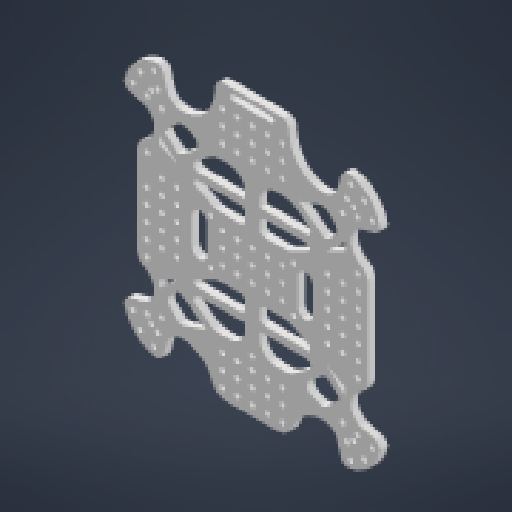
# Autodesk Inventor part: bottom
Saved by Autodesk Inventor 2023 (Build 270158000, 158)
## iProperties
Created: 2022-05-28
Part Number: bottom
Material: Generic
Document SubType Name: Modeling
Designer: vibhu
Density: 1 g/cm^3
Appearance: Default
Author: vibhu
Autodesk Inventor part; units mm, degrees
ref_plane "YZ Plane" through (0, 0, 0) normal (1, 0, 0) x (0, 1, 0)
ref_plane "XZ Plane" through (0, 0, 0) normal (0, 1, 0) x (-1, 0, 0)
ref_plane "XY Plane" through (0, 0, 0) normal (0, 0, 1) x (1, 0, 0)
sketch "Base Sketch With Dimensions" plane through (0, 0, 0) normal (0, 0, 1) x (1, 0, 0)
  circle A0 centre (74.1421, 4.1421) radius 1.75
  circle A1 centre (60, -10) radius 1.75
  circle A2 centre (69.6593, -7.4118) radius 1.75
  circle A3 centre (79.3185, -4.8236) radius 1.75
  circle A4 centre (65.1764, 9.3185) radius 1.75
  circle A5 centre (62.5882, -0.3407) radius 1.75
  line L0 (65.1764, 9.3185) -> (60, -10) construction
  line L1 (60, -10) -> (74.1421, 4.1421) construction
  line L2 (60, -10) -> (79.3185, -4.8236) construction
  circle A6 centre (67.0711, -2.9289) radius 1.75
  circle A7 centre (-74.1421, -144.1421) radius 1.75
  circle A8 centre (-60, -130) radius 1.75
  circle A9 centre (-69.6593, -132.5882) radius 1.75
  circle A10 centre (-79.3185, -135.1764) radius 1.75
  circle A11 centre (-65.1764, -149.3185) radius 1.75
  circle A12 centre (-62.5882, -139.6593) radius 1.75
  line L3 (-65.1764, -149.3185) -> (-60, -130) construction
  line L4 (-60, -130) -> (-74.1421, -144.1421) construction
  line L5 (-60, -130) -> (-79.3185, -135.1764) construction
  circle A13 centre (-67.0711, -137.0711) radius 1.75
  circle A14 centre (-74.1421, 4.1421) radius 1.75
  circle A15 centre (-60, -10) radius 1.75
  circle A16 centre (-62.5882, -0.3407) radius 1.75
  circle A17 centre (-65.1764, 9.3185) radius 1.75
  circle A18 centre (-79.3185, -4.8236) radius 1.75
  circle A19 centre (-69.6593, -7.4118) radius 1.75
  line L6 (-79.3185, -4.8236) -> (-60, -10) construction
  line L7 (-60, -10) -> (-74.1421, 4.1421) construction
  line L8 (-60, -10) -> (-65.1764, 9.3185) construction
  circle A20 centre (-67.0711, -2.9289) radius 1.75
  circle A21 centre (74.1421, -144.1421) radius 1.75
  circle A22 centre (60, -130) radius 1.75
  circle A23 centre (62.5882, -139.6593) radius 1.75
  circle A24 centre (65.1764, -149.3185) radius 1.75
  circle A25 centre (79.3185, -135.1764) radius 1.75
  circle A26 centre (69.6593, -132.5882) radius 1.75
  line L9 (79.3185, -135.1764) -> (60, -130) construction
  line L10 (60, -130) -> (74.1421, -144.1421) construction
  line L11 (60, -130) -> (65.1764, -149.3185) construction
  circle A27 centre (67.0711, -137.0711) radius 1.75
  line L12 (-22.5, 0) -> (22.5, 0) construction
  line L13 (22.5, 0) -> (22.5, -140) construction
  line L14 (22.5, -140) -> (-22.5, -140) construction
  line L15 (-22.5, -140) -> (-22.5, 0) construction
  line L16 (-67.5, -35) -> (-42.5, -35) construction
  line L17 (-42.5, -35) -> (-42.5, -105) construction
  line L18 (-42.5, -105) -> (-67.5, -105) construction
  line L19 (-67.5, -105) -> (-67.5, -35) construction
  line L20 (42.5, -35) -> (67.5, -35) construction
  line L21 (67.5, -35) -> (67.5, -105) construction
  line L22 (67.5, -105) -> (42.5, -105) construction
  line L23 (42.5, -105) -> (42.5, -35) construction
  line L24 (-42.5, -70) -> (-22.5, -70) construction
  line L25 (22.5, -70) -> (42.5, -70) construction
  line L26 (-60, -10) -> (-60, -130) construction
  line L27 (60, -130) -> (-60, -130) construction
  arc A28 (84.5585, -5.3225) -> (64.6775, 14.5585) centre (60, -10) ccw
  line L28 (58.9124, 10.9409) -> (54.7169, -4.7169)
  line L29 (80.9409, -11.0876) -> (65.2831, -15.2831)
  arc A29 (64.6775, 14.5585) -> (58.9124, 10.9409) centre (63.742, 9.6468) ccw
  arc A30 (80.9409, -11.0876) -> (84.5585, -5.3225) centre (79.6468, -6.258) ccw
  line L30 (0, 57.9218) -> (0, -169.8921) construction
  line L31 (161.6421, -70) -> (-111.9125, -70) construction
  arc A31 (-64.6775, 14.5585) -> (-84.5585, -5.3225) centre (-60, -10) ccw
  line L32 (-58.9124, 10.9409) -> (-54.7169, -4.7169)
  line L33 (-80.9409, -11.0876) -> (-65.2831, -15.2831)
  arc A32 (-58.9124, 10.9409) -> (-64.6775, 14.5585) centre (-63.742, 9.6468) ccw
  arc A33 (-84.5585, -5.3225) -> (-80.9409, -11.0876) centre (-79.6468, -6.258) ccw
  arc A34 (64.6775, -154.5585) -> (84.5585, -134.6775) centre (60, -130) ccw
  line L34 (58.9124, -150.9409) -> (54.7169, -135.2831)
  line L35 (80.9409, -128.9124) -> (65.2831, -124.7169)
  arc A35 (58.9124, -150.9409) -> (64.6775, -154.5585) centre (63.742, -149.6468) ccw
  arc A36 (84.5585, -134.6775) -> (80.9409, -128.9124) centre (79.6468, -133.742) ccw
  arc A37 (-64.6775, -154.5585) -> (-58.9124, -150.9409) centre (-63.742, -149.6468) ccw
  line L36 (-58.9124, -150.9409) -> (-54.7169, -135.2831)
  arc A38 (-84.5585, -134.6775) -> (-64.6775, -154.5585) centre (-60, -130) ccw
  arc A39 (-80.9409, -128.9124) -> (-84.5585, -134.6775) centre (-79.6468, -133.742) ccw
  line L37 (-80.9409, -128.9124) -> (-65.2831, -124.7169)
  line L38 (54.7169, -4.7169) -> (65.2831, -15.2831) construction
  line L39 (-65.2831, -15.2831) -> (-65.2831, -124.7169)
  line L40 (65.2831, -124.7169) -> (65.2831, -15.2831)
  line L41 (-54.7169, -4.7169) -> (54.7169, -4.7169)
  line L42 (-54.7169, -135.2831) -> (54.7169, -135.2831)
  point P0 (-42.5, -70)
  point P1 (0, -130)
  point P2 (0, -140)
  point P3 (-60, -70)
  point P4 (0, 0)
  point P5 (0, 0)
  point P6 (-67.5, -70)
  point P7 (85, -10)
  point P8 (60, 15)
  point P9 (42.5, -70)
  dimension "d0" = 3.5
  dimension "d1" = 30
  dimension "d2" = 30
  dimension "d3" = 20
  dimension "d5" = 30
  dimension "d6" = 30
  dimension "d9" = 30
  dimension "d10" = 30
  dimension "d13" = 30
  dimension "d14" = 30
  dimension "d16" = 45
  dimension "d17" = 140
  dimension "d18" = 25
  dimension "d19" = 70
  dimension "d23" = 135
  dimension "d25" = 135
  dimension "d29" = 20
  dimension "d30" = 120
  dimension "d32" = 120
  dimension "d40" = 25
  dimension "d41" = 5
  constraints: 86 end point, 40 centre point, 28 equal radius, 27 symmetric about line, 26 point on circle, 25 midpoint, 18 coincident, 14 equal length, 10 horizontal alignment, 9 parallel, 7 perpendicular, 5 point on line, 4 horizontal, 4 tangent, 4 vertical alignment, 3 vertical, 10 other
  measures "d0" diameter of A4
  measures "d1" angle of L1 L0
  measures "d2" angle of L2 L1
  measures "d3" distance of L0.end L2.end
  measures "d5" angle of L4 L3
  measures "d6" angle of L5 L4
  measures "d9" angle of L7 L6
  measures "d10" angle of L8 L7
  measures "d13" angle of L10 L9
  measures "d14" angle of L11 L10
  measures "d16" distance of L13.end L14.end
  measures "d17" distance of L12.end L13.end
  measures "d18" distance of L16.start L16.end
  measures "d19" distance of L18.end L16.start
  measures "d23" angle of L26 L4
  measures "d25" angle of L26 L7
  measures "d29" distance between parallel lines of L15 L17
  measures "d30" distance of point (60, -10) point (-60, -10)
  measures "d32" distance of L6.end L3.end
  measures "d40" radius of A28
  measures "d41" radius of A29
extrude "Extrusion1" add sketch "Base Sketch With Dimensions" along normal blind 5
fillet "Fillet1" radius 10 8 edges at (54.7169, -135.2831, 2.5) (-54.7169, -135.2831, 2.5) (-65.2831, -124.7169, 2.5) (-65.2831, -15.2831, 2.5) (54.7169, -4.7169, 2.5) (-54.7169, -4.7169, 2.5) (65.2831, -15.2831, 2.5) (65.2831, -124.7169, 2.5)
sketch "Sketch3" plane through (0, 0, 0) normal (0, 0, -1) x (-1, 0, 0)
  circle A0 centre (70, -50) radius 1.75
  line L0 (0, 0) -> (-18.5117, 0) construction
  line L1 (0, 0) -> (0, -12.0208) construction
  line L2 (-65.2831, -117.0436) -> (-65.2831, -22.9564) construction
  line L3 (-47.0436, -4.7169) -> (47.0436, -4.7169) construction
  line L4 (84.7487, 0.6066) -> (70.6066, 14.7487) construction
  line L5 (-70.6066, 14.7487) -> (-84.7487, 0.6066) construction
  line L6 (-84.7487, -140.6066) -> (-70.6066, -154.7487) construction
  line L7 (70.6066, -154.7487) -> (84.7487, -140.6066) construction
  line L8 (-65.2831, -22.9564) -> (-65.2831, -117.0436) construction
  line L9 (-84.7487, 0.6066) -> (-70.6066, 14.7487) construction
  circle A1 centre (20, -150) radius 1.75
  circle A2 centre (10, -150) radius 1.75
  circle A3 centre (0, -150) radius 1.75
  circle A4 centre (-10, -150) radius 1.75
  circle A5 centre (-20, -150) radius 1.75
  circle A6 centre (20, -140) radius 1.75
  circle A7 centre (10, -140) radius 1.75
  circle A8 centre (0, -140) radius 1.75
  circle A9 centre (-10, -140) radius 1.75
  circle A10 centre (-20, -140) radius 1.75
  circle A11 centre (20, -130) radius 1.75
  circle A12 centre (10, -130) radius 1.75
  circle A13 centre (0, -130) radius 1.75
  circle A14 centre (-10, -130) radius 1.75
  circle A15 centre (-20, -130) radius 1.75
  line L10 (3.2457, -70) -> (-3.2457, -70) construction
  circle A16 centre (20, 10) radius 1.75
  circle A17 centre (10, 10) radius 1.75
  circle A18 centre (0, 10) radius 1.75
  circle A19 centre (-10, 10) radius 1.75
  circle A20 centre (-20, 10) radius 1.75
  circle A21 centre (20, 0) radius 1.75
  circle A22 centre (10, 0) radius 1.75
  circle A23 centre (0, 0) radius 1.75
  circle A24 centre (-10, 0) radius 1.75
  circle A25 centre (-20, 0) radius 1.75
  circle A26 centre (20, -10) radius 1.75
  circle A27 centre (10, -10) radius 1.75
  circle A28 centre (0, -10) radius 1.75
  circle A29 centre (-10, -10) radius 1.75
  circle A30 centre (-20, -10) radius 1.75
  circle A31 centre (20, -80) radius 1.75
  circle A32 centre (10, -80) radius 1.75
  circle A33 centre (0, -80) radius 1.75
  circle A34 centre (-10, -80) radius 1.75
  circle A35 centre (-20, -80) radius 1.75
  circle A36 centre (20, -70) radius 1.75
  circle A37 centre (10, -70) radius 1.75
  circle A38 centre (0, -70) radius 1.75
  circle A39 centre (-10, -70) radius 1.75
  circle A40 centre (-20, -70) radius 1.75
  circle A41 centre (20, -60) radius 1.75
  circle A42 centre (10, -60) radius 1.75
  circle A43 centre (0, -60) radius 1.75
  circle A44 centre (-10, -60) radius 1.75
  circle A45 centre (-20, -60) radius 1.75
  line L11 (47.0436, -135.2831) -> (-47.0436, -135.2831) projected
  circle A46 centre (60, -50) radius 1.75
  circle A47 centre (50, -50) radius 1.75
  circle A48 centre (70, -60) radius 1.75
  circle A49 centre (60, -60) radius 1.75
  circle A50 centre (50, -60) radius 1.75
  circle A51 centre (70, -70) radius 1.75
  circle A52 centre (60, -70) radius 1.75
  circle A53 centre (50, -70) radius 1.75
  circle A54 centre (70, -80) radius 1.75
  circle A55 centre (60, -80) radius 1.75
  circle A56 centre (50, -80) radius 1.75
  circle A57 centre (70, -90) radius 1.75
  circle A58 centre (60, -90) radius 1.75
  circle A59 centre (50, -90) radius 1.75
  circle A60 centre (-70, -50) radius 1.75
  circle A61 centre (-60, -50) radius 1.75
  circle A62 centre (-50, -50) radius 1.75
  circle A63 centre (-70, -60) radius 1.75
  circle A64 centre (-60, -60) radius 1.75
  circle A65 centre (-50, -60) radius 1.75
  circle A66 centre (-70, -70) radius 1.75
  circle A67 centre (-60, -70) radius 1.75
  circle A68 centre (-50, -70) radius 1.75
  circle A69 centre (-70, -80) radius 1.75
  circle A70 centre (-60, -80) radius 1.75
  circle A71 centre (-50, -80) radius 1.75
  circle A72 centre (-70, -90) radius 1.75
  circle A73 centre (-60, -90) radius 1.75
  circle A74 centre (-50, -90) radius 1.75
  line L12 (65.2831, -22.9564) -> (65.2831, -117.0436) projected
  point P0 (0, -227.282)
  point P1 (0, 87.282)
  point P2 (0, -135.2831)
  point P3 (65.2831, -70)
  dimension "d82" = 10
  dimension "d85" = 10
  dimension "d90" = 10
  dimension "d93" = 10
  dimension "d229" = 50
  dimension "d232" = 10
  dimension "d235" = 10
  dimension "d238" = 3.5
  dimension "d239" = 100
  constraints: 75 centre point, 32 symmetric about line, 10 end point, 4 horizontal, 4 vertical, 3 midpoint, 2 equal radius, 2 horizontal alignment, 2 vertical alignment, 1 coincident, 114 other
  measures "d82" distance of A1.centre A2.centre
  measures "d85" distance of A1.centre A6.centre
  measures "d90" distance of A31.centre A32.centre
  measures "d93" distance of A31.centre A36.centre
  measures "d229" distance of A13.centre A33.centre
  measures "d232" distance of A0.centre A46.centre
  measures "d235" distance of A0.centre A48.centre
  measures "d238" diameter of A0
  measures "d239" distance of A68.centre A53.centre
sketch "Sketch4" plane through (0, 0, 0) normal (0, 0, -1) x (-1, 0, 0)
  line L0 (-65.2831, -117.0436) -> (-65.2831, -22.9564) projected
  line L1 (65.2831, -22.9564) -> (65.2831, -117.0436) construction
  line L2 (76.75, -105) -> (76.75, -35)
  line L3 (-76.75, -105) -> (-76.75, -35)
  line L4 (25, 15) -> (-25, 15)
  line L5 (25, -156.75) -> (-25, -156.75)
  line L6 (-47.0436, -4.7169) -> (47.0436, -4.7169) projected
  line L7 (47.0436, -135.2831) -> (-47.0436, -135.2831) projected
  arc A0 (76.75, -105) -> (65.2831, -117.0436) centre (77.3412, -117.0436) ccw
  arc A1 (65.2831, -22.9564) -> (76.75, -35) centre (77.3412, -22.9564) ccw
  line L8 (-65.2831, -117.0436) -> (-65.2831, -22.9564) projected
  arc A2 (-76.75, -35) -> (-65.2831, -22.9564) centre (-77.3412, -22.9564) ccw
  arc A3 (-65.2831, -117.0436) -> (-76.75, -105) centre (-77.3412, -117.0436) ccw
  line L9 (47.0436, -135.2831) -> (-47.0436, -135.2831) projected
  arc A4 (-25, -156.75) -> (-47.0436, -135.2831) centre (-47.0436, -157.3345) ccw
  arc A5 (47.0436, -135.2831) -> (25, -156.75) centre (47.0436, -157.3345) ccw
  arc A6 (25, 15) -> (47.0436, -4.7169) centre (47.0436, 17.464) ccw
  arc A7 (-56.7029, 2.6949) -> (-47.0436, -4.7169) centre (-47.0436, 5.2831) ccw construction
  arc A8 (-47.0436, -4.7169) -> (-25, 15) centre (-47.0436, 17.464) ccw
  circle A9 centre (0, -150) radius 1.75 projected
  circle A10 centre (0, 10) radius 1.75 projected
  circle A11 centre (70, -70) radius 1.75 projected
  circle A12 centre (-70, -70) radius 1.75 projected
  line L10 (65.2831, -22.9564) -> (65.2831, -117.0436) projected
  line L11 (23.8822, 25) -> (-23.8822, 25)
  line L12 (23.8822, 25) -> (25, 15)
  line L13 (-23.8822, 25) -> (-25, 15)
  line L14 (12.5, 20) -> (-12.5, 20) construction
  line L15 (12.5, 22) -> (-12.5, 22)
  line L16 (-12.5, 18) -> (12.5, 18)
  arc A13 (12.5, 18) -> (12.5, 22) centre (12.5, 20) ccw
  arc A14 (-12.5, 22) -> (-12.5, 18) centre (-12.5, 20) ccw
  point P0 (0, 0)
  point P1 (0, 15)
  point P2 (0, -4.7169)
  point P3 (0, -156.75)
  point P4 (0, -135.2831)
  point P5 (-76.75, -70)
  point P6 (-65.2831, -70)
  point P7 (65.2831, -70)
  point P8 (76.75, -70)
  point P9 (0, 20)
  point P10 (0, -4.7169)
  point P11 (24.4411, 20)
  dimension "d97" = 5
  dimension "d98" = 50
  dimension "d106" = 70
  dimension "d240" = 5
  dimension "d241" = 5
  dimension "d242" = 5
  dimension "d244" = 4
  dimension "d246" = 25
  dimension "d247" = 10
  constraints: 22 end point, 20 point on circle, 14 tangent, 10 centre point, 10 midpoint, 4 horizontal, 4 horizontal alignment, 3 parallel, 3 vertical alignment, 2 vertical
  measures "d97" distance edge to line of A9 L5
  measures "d98" distance of L5.start L5.end
  measures "d106" distance of L2.start L2.end
  measures "d240" distance from line of A10.centre L4
  measures "d241" distance edge to line of A12 L3
  measures "d242" distance edge to line of A11 L2
  measures "d244" diameter of A14
  measures "d246" distance of L14.start L14.end
  measures "d247" distance between parallel lines of L11 L4
extrude "Side Extensions" add sketch "Sketch4" against normal up to surface (5 mm away) contours A3 L3 A2 L0 | A0 L10 A1 L2 | A6 L6 A8 L4 | L4 L13 L11 L12 | L5 A4 L7 A5 | A12
extrude "Bottom Holes" cut sketch "Sketch3" against normal up to surface (5 mm away) contours A1 | A2 | A3 | A4 | A5 | A6 | A7 | A8 | A9 | A10 | A11 | A12 | A13 | A14 | A15 | A16 | A17 | A18 | A19 | A20 | A21 | A22 | A23 | A24 | A25 | A26 | A27 | A28 | A29 | A30 | A31 | A32 | A33 | A34 | A35 | A36 | A37 | A38 | A39 | A40 | A41 | A42 | A43 | A44 | A45 | A46 | A47 | A48 | A49 | A50 | A51 | A52 | A53 | A54 | A55 | A56 | A57 | A58 | A59 | A60 | A61 | A62 | A63 | A64 | A65 | A66 | A67 | A68 | A69 | A70 | A71 | A72 | A73 | A74
fillet "Fillet2" radius 10 8 edges at (-76.75, -35, 2.5) (-76.75, -105, 2.5) (76.75, -105, 2.5) (76.75, -35, 2.5) (-25, 15, 2.5) (25, 15, 2.5) (25, -156.75, 2.5) (-25, -156.75, 2.5)
sketch "Sketch6" plane through (0, 0, 0) normal (0, 0, -1) x (-1, 0, 0)
  line L0 (-42.5, -35) -> (-67.5, -35) construction
  line L1 (-42.5, -105) -> (-42.5, -35) construction
  line L2 (-67.5, -35) -> (-67.5, -105) construction
  line L3 (-67.5, -105) -> (-42.5, -105) construction
  line L4 (42.5, -105) -> (67.5, -105) construction
  line L5 (42.5, -35) -> (42.5, -105) construction
  line L6 (67.5, -105) -> (67.5, -35) construction
  line L7 (67.5, -35) -> (42.5, -35) construction
  line L8 (22.5, -140) -> (22.5, 0) construction
  line L9 (22.5, 0) -> (-22.5, 0) construction
  line L10 (-22.5, 0) -> (-22.5, -140) construction
  line L11 (-22.5, -140) -> (22.5, -140) construction
  circle A0 centre (-69.75, -40) radius 1.75
  circle A1 centre (-69.75, -100) radius 1.75
  circle A2 centre (69.75, -40) radius 1.75
  circle A3 centre (69.75, -100) radius 1.75
  point P0 (0, 0)
  point P1 (0, 0)
  point P2 (67.5, -70)
  dimension "d134" = 3.5
  dimension "d135" = 0.5
  dimension "d136" = 0.5
  dimension "d137" = 30
  dimension "d138" = 30
  constraints: 4 centre point, 3 equal radius, 2 horizontal alignment, 2 vertical alignment, 1 midpoint
  measures "d134" diameter of A0
  measures "d135" distance edge to line of A1 L2
  measures "d136" distance edge to line of A3 L6
  measures "d137" vertical distance of point (67.5, -70) A2.centre
  measures "d138" vertical distance of point (67.5, -70) A3.centre
extrude "ESC holders" cut sketch "Sketch6" against normal up to surface (5 mm away)
sketch "Sketch7" plane through (0, 0, 0) normal (0, 0, -1) x (-1, 0, 0)
  circle A0 centre (-20, 10) radius 3.25
  circle A1 centre (50, -50) radius 3.25
  circle A2 centre (-20, -60) radius 3.25
  circle A3 centre (-70, -50) radius 3.25
  circle A4 centre (-20, -130) radius 3.25
  circle A5 centre (-20, 10) radius 1.75 construction
  circle A6 centre (-20, -60) radius 1.75 construction
  circle A7 centre (-20, -130) radius 1.75 construction
  line L0 (0, 0) -> (10.4929, 0) construction
  line L1 (0, 0) -> (0, -9.7144) construction
  circle A8 centre (-10, 10) radius 3.25
  circle A9 centre (0, 10) radius 3.25
  circle A10 centre (10, 10) radius 3.25
  circle A11 centre (20, 10) radius 3.25
  circle A12 centre (-20, 0) radius 3.25
  circle A13 centre (-10, 0) radius 3.25
  circle A14 centre (0, 0) radius 3.25
  circle A15 centre (10, 0) radius 3.25
  circle A16 centre (20, 0) radius 3.25
  circle A17 centre (-20, -10) radius 3.25
  circle A18 centre (-10, -10) radius 3.25
  circle A19 centre (0, -10) radius 3.25
  circle A20 centre (10, -10) radius 3.25
  circle A21 centre (20, -10) radius 3.25
  circle A22 centre (-60, -50) radius 3.25
  circle A23 centre (-50, -50) radius 3.25
  circle A24 centre (-70, -60) radius 3.25
  circle A25 centre (-60, -60) radius 3.25
  circle A26 centre (-50, -60) radius 3.25
  circle A27 centre (-70, -70) radius 3.25
  circle A28 centre (-60, -70) radius 3.25
  circle A29 centre (-50, -70) radius 3.25
  circle A30 centre (-70, -80) radius 3.25
  circle A31 centre (-60, -80) radius 3.25
  circle A32 centre (-50, -80) radius 3.25
  circle A33 centre (-70, -90) radius 3.25
  circle A34 centre (-60, -90) radius 3.25
  circle A35 centre (-50, -90) radius 3.25
  circle A36 centre (-10, -60) radius 3.25
  circle A37 centre (0, -60) radius 3.25
  circle A38 centre (10, -60) radius 3.25
  circle A39 centre (20, -60) radius 3.25
  circle A40 centre (-20, -70) radius 3.25
  circle A41 centre (-10, -70) radius 3.25
  circle A42 centre (0, -70) radius 3.25
  circle A43 centre (10, -70) radius 3.25
  circle A44 centre (20, -70) radius 3.25
  circle A45 centre (-20, -80) radius 3.25
  circle A46 centre (-10, -80) radius 3.25
  circle A47 centre (0, -80) radius 3.25
  circle A48 centre (10, -80) radius 3.25
  circle A49 centre (20, -80) radius 3.25
  circle A50 centre (60, -50) radius 3.25
  circle A51 centre (70, -50) radius 3.25
  circle A52 centre (50, -60) radius 3.25
  circle A53 centre (60, -60) radius 3.25
  circle A54 centre (70, -60) radius 3.25
  circle A55 centre (50, -70) radius 3.25
  circle A56 centre (60, -70) radius 3.25
  circle A57 centre (70, -70) radius 3.25
  circle A58 centre (50, -80) radius 3.25
  circle A59 centre (60, -80) radius 3.25
  circle A60 centre (70, -80) radius 3.25
  circle A61 centre (50, -90) radius 3.25
  circle A62 centre (60, -90) radius 3.25
  circle A63 centre (70, -90) radius 3.25
  circle A64 centre (-10, -130) radius 3.25
  circle A65 centre (0, -130) radius 3.25
  circle A66 centre (10, -130) radius 3.25
  circle A67 centre (20, -130) radius 3.25
  circle A68 centre (-20, -140) radius 3.25
  circle A69 centre (-10, -140) radius 3.25
  circle A70 centre (0, -140) radius 3.25
  circle A71 centre (10, -140) radius 3.25
  circle A72 centre (20, -140) radius 3.25
  circle A73 centre (-20, -150) radius 3.25
  circle A74 centre (-10, -150) radius 3.25
  circle A75 centre (0, -150) radius 3.25
  circle A76 centre (10, -150) radius 3.25
  circle A77 centre (20, -150) radius 3.25
  dimension "d151" = 6.5
  dimension "d154" = 10
  dimension "d157" = 10
  dimension "d162" = 10
  dimension "d165" = 10
  dimension "d170" = 10
  dimension "d173" = 10
  dimension "d178" = 10
  dimension "d181" = 10
  dimension "d186" = 10
  dimension "d189" = 10
  constraints: 75 centre point, 6 horizontal, 6 vertical, 4 end point, 4 equal radius, 3 concentric, 2 coincident, 140 other
  measures "d151" diameter of A0
  measures "d154" distance of A0.centre A8.centre
  measures "d157" distance of A0.centre A12.centre
  measures "d162" distance of A3.centre A22.centre
  measures "d165" distance of A3.centre A24.centre
  measures "d170" distance of A2.centre A36.centre
  measures "d173" distance of A2.centre A40.centre
  measures "d178" distance of A1.centre A50.centre
  measures "d181" distance of A1.centre A52.centre
  measures "d186" distance of A4.centre A64.centre
  measures "d189" distance of A4.centre A68.centre
extrude "Hole Countersinks" cut sketch "Sketch7" against normal blind 2
sketch "Skeleton Sketch" plane through (0, 0, 0) normal (0, 0, -1) x (-1, 0, 0)
  line L0 (-25, -55) -> (25, -55)
  line L1 (25, -55) -> (25, -85)
  line L2 (25, -85) -> (-25, -85)
  line L3 (-25, -85) -> (-25, -55)
  circle A0 centre (0, -70) radius 1.75 construction
  line L4 (-25, -55) -> (25, -85) construction
  line L5 (25, -55) -> (-25, -85) construction
  line L6 (-25, 15) -> (25, 15)
  line L7 (25, 15) -> (25, -15)
  line L8 (25, -15) -> (-25, -15)
  line L9 (-25, -15) -> (-25, 15)
  circle A1 centre (0, 0) radius 1.75 construction
  line L10 (-25, 15) -> (25, -15) construction
  line L11 (25, 15) -> (-25, -15) construction
  line L12 (-25, -125) -> (25, -125)
  line L13 (25, -125) -> (25, -155)
  line L14 (25, -155) -> (-25, -155)
  line L15 (-25, -155) -> (-25, -125)
  line L16 (-25, -125) -> (25, -155) construction
  line L17 (25, -125) -> (-25, -155) construction
  circle A2 centre (0, -140) radius 1.75 construction
  line L18 (-75, -45) -> (-45, -45)
  line L19 (-45, -45) -> (-45, -95)
  line L20 (-45, -95) -> (-75, -95)
  line L21 (-75, -95) -> (-75, -45)
  line L22 (-75, -45) -> (-45, -95) construction
  line L23 (-45, -45) -> (-75, -95) construction
  line L24 (45, -45) -> (75, -45)
  line L25 (75, -45) -> (75, -95)
  line L26 (75, -95) -> (45, -95)
  line L27 (45, -95) -> (45, -45)
  line L28 (45, -45) -> (75, -95) construction
  line L29 (75, -45) -> (45, -95) construction
  line L30 (0, -15) -> (0, -55)
  line L31 (0, -55) -> (0, -15)
  line L32 (0, -85) -> (0, -125) construction
  line L33 (-45, -45) -> (-25, -55)
  line L34 (-45, -95) -> (-25, -85)
  line L35 (25, -55) -> (45, -45)
  line L36 (45, -95) -> (25, -85)
  line L37 (-40, -53.0902) -> (-40, -86.9098)
  line L38 (-40, -86.9098) -> (-30, -81.9098)
  line L39 (-30, -81.9098) -> (-30, -58.0902)
  line L40 (-30, -58.0902) -> (-40, -53.0902)
  line L41 (40, -53.0902) -> (40, -86.9098)
  line L42 (40, -86.9098) -> (30, -81.9098)
  line L43 (30, -81.9098) -> (30, -58.0902)
  line L44 (30, -58.0902) -> (40, -53.0902)
  line L45 (-25, -70) -> (25, -70) construction
  line L46 (45, -39.4098) -> (23.8197, -50)
  line L47 (23.8197, -50) -> (-23.8197, -50)
  line L48 (-23.8197, -50) -> (-45, -39.4098)
  line L49 (-45, -39.4098) -> (45, -39.4098)
  line L50 (45, -100.5902) -> (23.8197, -90)
  line L51 (23.8197, -90) -> (-23.8197, -90)
  line L52 (-23.8197, -90) -> (-45, -100.5902)
  line L53 (-45, -100.5902) -> (45, -100.5902)
  line L54 (45, -105.5902) -> (25, -120)
  line L55 (25, -120) -> (5, -120)
  line L56 (5, -120) -> (5, -105.5902)
  line L57 (5, -105.5902) -> (45, -105.5902)
  line L58 (5, -105.5902) -> (5, -100.5902)
  line L59 (60, -130) -> (74.1421, -144.1421) construction
  line L60 (47.6256, -128.2322) -> (30.6833, -122.0678)
  line L61 (30.6833, -122.0678) -> (48.7806, -109.0289)
  line L62 (48.7806, -109.0289) -> (58.2322, -117.6256)
  line L63 (58.2322, -117.6256) -> (47.6256, -128.2322)
  line L64 (61.7717, -114.0861) -> (49.2946, -102.7375)
  line L65 (49.2946, -102.7375) -> (61.7717, -108.976)
  line L66 (61.7717, -108.976) -> (61.7717, -114.0861)
  arc A3 (71.5515, -106.4664) -> (65.2831, -117.0436) centre (77.3412, -117.0436) ccw construction
  line L67 (25, -70) -> (-25, -70) construction
  line L68 (-45, -105.5902) -> (-25, -120)
  line L69 (-25, -120) -> (-5, -120)
  line L70 (-5, -120) -> (-5, -105.5902)
  line L71 (-5, -105.5902) -> (-45, -105.5902)
  line L72 (-5, -105.5902) -> (-5, -100.5902)
  line L73 (-47.6256, -128.2322) -> (-30.6833, -122.0678)
  line L74 (-30.6833, -122.0678) -> (-48.7806, -109.0289)
  line L75 (-48.7806, -109.0289) -> (-58.2322, -117.6256)
  line L76 (-58.2322, -117.6256) -> (-47.6256, -128.2322)
  line L77 (-61.7717, -114.0861) -> (-49.2946, -102.7375)
  line L78 (-49.2946, -102.7375) -> (-61.7717, -108.976)
  line L79 (-61.7717, -108.976) -> (-61.7717, -114.0861)
  line L80 (45, -34.4098) -> (25, -20)
  line L81 (25, -20) -> (5, -20)
  line L82 (5, -20) -> (5, -34.4098)
  line L83 (5, -34.4098) -> (45, -34.4098)
  line L84 (5, -34.4098) -> (5, -39.4098)
  line L85 (47.6256, -11.7678) -> (30.6833, -17.9322)
  line L86 (30.6833, -17.9322) -> (48.7806, -30.9711)
  line L87 (48.7806, -30.9711) -> (58.2322, -22.3744)
  line L88 (58.2322, -22.3744) -> (47.6256, -11.7678)
  line L89 (61.7717, -25.9139) -> (49.2946, -37.2625)
  line L90 (49.2946, -37.2625) -> (61.7717, -31.024)
  line L91 (61.7717, -31.024) -> (61.7717, -25.9139)
  line L92 (-47.6256, -11.7678) -> (-30.6833, -17.9322)
  line L93 (-30.6833, -17.9322) -> (-48.7806, -30.9711)
  line L94 (-48.7806, -30.9711) -> (-58.2322, -22.3744)
  line L95 (-58.2322, -22.3744) -> (-47.6256, -11.7678)
  line L96 (-61.7717, -25.9139) -> (-49.2946, -37.2625)
  line L97 (-61.7717, -31.024) -> (-61.7717, -25.9139)
  line L98 (-49.2946, -37.2625) -> (-61.7717, -31.024)
  line L99 (-5, -34.4098) -> (-45, -34.4098)
  line L100 (-45, -34.4098) -> (-25, -20)
  line L101 (-25, -20) -> (-5, -20)
  line L102 (-5, -20) -> (-5, -34.4098)
  line L103 (-5, -34.4098) -> (-5, -39.4098)
  circle A4 centre (60, -70) radius 1.75 construction
  circle A5 centre (-60, -70) radius 1.75 construction
  line L104 (-5, -39.4098) -> (-5, -50)
  line L105 (5, -39.4098) -> (5, -50)
  line L106 (5, -100.5902) -> (5, -90)
  line L107 (-5, -100.5902) -> (-5, -90)
  point P0 (0, 0)
  point P1 (0, -140)
  point P2 (60, -70)
  point P3 (0, -50)
  point P4 (0, -39.4098)
  point P5 (52.9289, -122.9289)
  point P6 (53.5064, -113.3272)
  point P7 (69.6467, -102.3499)
  dimension "d108" = 50
  dimension "d109" = 30
  dimension "d204" = 5
  dimension "d205" = 5
  dimension "d206" = 5
  dimension "d207" = 5
  dimension "d211" = 5
  dimension "d212" = 5
  dimension "d216" = 5
  dimension "d217" = 5
  dimension "d218" = 5
  dimension "d220" = 5
  dimension "d221" = 10
  dimension "d222" = 15
  dimension "d223" = 5
  constraints: 216 end point, 46 symmetric about line, 20 point on line, 19 midpoint, 18 parallel, 12 perpendicular, 8 equal length, 7 horizontal, 5 vertical alignment, 3 vertical, 2 coincident, 2 collinear
  measures "d108" distance of L1.end L2.end
  measures "d109" distance of L0.end L1.end
  measures "d204" distance between parallel lines of L19 L37
  measures "d205" distance between parallel lines of L33 L40
  measures "d206" distance between parallel lines of L39 L3
  measures "d207" distance between parallel lines of L34 L38
  measures "d211" distance between parallel lines of L0 L47
  measures "d212" distance between parallel lines of L35 L46
  measures "d216" distance between parallel lines of L32 L56
  measures "d217" distance between parallel lines of L53 L57
  measures "d218" distance between parallel lines of L12 L55
  measures "d220" distance between parallel lines of L54 L61
  measures "d221" distance from line of L63 L59.start
  measures "d222" distance of L62.end L60.start
  measures "d223" distance from line of point (53.506, -113.327) L64
extrude "Skeleton" cut sketch "Skeleton Sketch" against normal up to surface (5 mm away) contours L104 L47 L48 L49 | L49 L46 L47 L105 | L40 L39 L38 L37 | L41 L42 L43 L44 | L53 L106 L51 L50 | L53 L52 L51 L107 | L54 L55 L56 L57 | L60 L61 L62 L63 | L64 L65 L66 | L71 L70 L69 L68 | L76 L75 L74 L73 | L79 L78 L77 | L83 L82 L81 L80 | L88 L87 L86 L85 | L91 L90 L89 | L92 L93 L94 L95 | L96 L98 L97 | L99 L100 L101 L102
fillet "Fillet3" radius 5 8 edges at (40, -53.0902, 2.5) (-30, -58.0902, 2.5) (30, -58.0902, 2.5) (-40, -53.0902, 2.5) (-40, -86.9098, 2.5) (-30, -81.9098, 2.5) (40, -86.9098, 2.5) (30, -81.9098, 2.5)
fillet "Fillet4" radius 2 4 edges at (-45, -39.4098, 2.5) (-45, -100.5902, 2.5) (45, -100.5902, 2.5) (45, -39.4098, 2.5)
fillet "Fillet5" radius 10 4 edges at (-23.8197, -50, 2.5) (23.8197, -50, 2.5) (-23.8197, -90, 2.5) (23.8197, -90, 2.5)
fillet "Fillet6" radius 5 8 edges at (47.6256, -11.7678, 2.5) (58.2322, -22.3744, 2.5) (-47.6256, -11.7678, 2.5) (-30.6833, -17.9322, 2.5) (-47.6256, -128.2322, 2.5) (-58.2322, -117.6256, 2.5) (30.6833, -122.0678, 2.5) (47.6256, -128.2322, 2.5)
fillet "Fillet8" radius 10 8 edges at (-5, -20, 2.5) (25, -20, 2.5) (5, -20, 2.5) (-25, -20, 2.5) (-25, -120, 2.5) (-5, -120, 2.5) (5, -120, 2.5) (25, -120, 2.5)
fillet "Fillet9" radius 3 8 edges at (-45, -34.4098, 2.5) (-48.7806, -30.9711, 2.5) (45, -34.4098, 2.5) (48.7806, -30.9711, 2.5) (48.7806, -109.0289, 2.5) (45, -105.5902, 2.5) (-45, -105.5902, 2.5) (-48.7806, -109.0289, 2.5)
fillet "Fillet10" radius 3 8 edges at (-5, -100.5902, 2.5) (-5, -90, 2.5) (5, -90, 2.5) (5, -100.5902, 2.5) (5, -50, 2.5) (5, -39.4098, 2.5) (-5, -39.4098, 2.5) (-5, -50, 2.5)
fillet "Fillet11" radius 5 2 edges at (-23.8822, 25, 2.5) (23.8822, 25, 2.5)
sketch "Sketch8" plane through (0, 0, 0) normal (0, 0, -1) x (-1, 0, 0)
  circle A0 centre (27.5, -55) radius 1.75
  circle A1 centre (27.5, -85) radius 1.75
  circle A2 centre (-27.5, -85) radius 1.75
  circle A3 centre (-27.5, -55) radius 1.75
  circle A4 centre (0, -122) radius 1.75
  line L0 (-161.6421, -70) -> (111.9125, -70) construction
  line L1 (0, 57.9218) -> (0, -169.8921) construction
  circle A5 centre (27.5, 15) radius 1.75
  circle A6 centre (-27.5, 15) radius 1.75
  line L2 (12.5, 18) -> (-12.5, 18) projected
  point P0 (0, 0)
  point P1 (0, -55.9852)
  dimension "d249" = 15
  dimension "d250" = 15
  dimension "d252" = 3.5
  dimension "d253" = 27.5
  dimension "d254" = 27.5
  dimension "d255" = 85
  dimension "d258" = 140
  constraints: 7 centre point, 6 equal radius, 4 vertical alignment, 3 horizontal alignment, 1 midpoint, 1 point on line
  measures "d249" distance from line of A1.centre L0
  measures "d250" distance from line of L0 A0.centre
  measures "d252" diameter of A1
  measures "d253" horizontal distance of point (0, -55.985) A0.centre
  measures "d254" distance from line of L1 A3.centre
  measures "d255" distance from line of L0 A6.centre
  measures "d258" distance from line of L2 A4.centre
extrude "Extrusion9" cut sketch "Sketch8" against normal up to surface (5 mm away)
equation "\"d2\" = d1"
equation "\"d5\" = d1"
equation "\"d6\" = d5"
equation "\"d9\" = d1"
equation "\"d10\" = d9"
equation "\"d13\" = d1"
equation "\"d14\" = d13"
body "Solid1"
